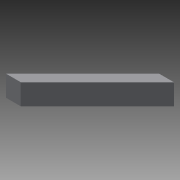
# Autodesk Inventor part: BallGuide2x4
Saved by Autodesk Inventor 2014 (Build 180170000, 170)
## iProperties
Created: 2016-02-06
Part Number: BallGuide2x4
Material: Generic
Document SubType Name: Modeling
Designer: choices
Density: 1 g/cm^3
Appearance: Default
Author: choices
Autodesk Inventor part; units mm, degrees
ref_plane "YZ Plane" through (0, 0, 0) normal (1, 0, 0) x (0, 1, 0)
ref_plane "XZ Plane" through (0, 0, 0) normal (0, 1, 0) x (-1, 0, 0)
ref_plane "XY Plane" through (0, 0, 0) normal (0, 0, 1) x (1, 0, 0)
sketch "Sketch1" plane through (0, 0, 0) normal (0, 1, 0) x (-1, 0, 0)
  line L0 (-75.001, -57.2471) -> (65.08, 82.8339)
  line L1 (-75.001, -57.2471) -> (123.1034, -57.2471) construction
  line L2 (-75.001, -57.2471) -> (-61.5307, -70.7175)
  line L3 (-61.5307, -70.7175) -> (92.0207, 82.8339)
  line L4 (92.0207, 82.8339) -> (65.08, 82.8339)
  line L5 (-75.001, -57.2471) -> (-48.0603, -57.2471)
  point P0 (0, 0)
  dimension "d0" = 45
  dimension "d1" = 140.081
  dimension "d2" = 19.05
  constraints: 12 end point, 2 perpendicular, 2 point on line, 1 equal length, 1 horizontal, 1 parallel
  measures "d0" angle of L1 L0
  measures "d1" horizontal distance of L0.end L0.start
  measures "d2" distance of L0.start L2.end
extrude "Extrusion1" add sketch "Sketch1" along normal blind 38.1 contours L0 L4 L3 L5
body "Solid1"
